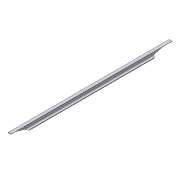
# Autodesk Inventor part: GE-12019-03
Saved by Autodesk Inventor 2012 (Build 160160000, 160)
## iProperties
Created: 2011-06-10
Part Number: GE-12019-03
Document SubType Name: Modeling
Designer: dfoster
Density: 2.71 g/cm^3
Material: Aluminum-6061
Mass: 4063.76 g
Surface Area: 9477.73 cm^2
Volume: 1499.54 cm^3
Description: Channel, Outside
Title: Channel, Outside
Author: dfoster
Autodesk Inventor part; units mm, degrees
ref_plane "YZ Plane" through (0, 0, 0) normal (1, 0, 0) x (0, 1, 0)
ref_plane "XZ Plane" through (0, 0, 0) normal (0, 1, 0) x (-1, 0, 0)
sketch "Sketch1" plane through (0, 0, 0) normal (0, 0, 1) x (1, 0, 0)
  line L0 (0, 0) -> (38.1, 0)
  line L1 (38.1, 76.2) -> (0, 76.2)
  line L2 (0, 76.2) -> (0, 0)
  line L3 (6.5532, 15.2924) -> (6.5532, 60.9076)
  line L4 (12.2838, 67.6723) -> (35.9776, 71.6213)
  line L5 (38.1, 76.2) -> (38.1, 74.1267)
  line L6 (12.2838, 8.5277) -> (35.9776, 4.5787)
  line L7 (38.1, 0) -> (38.1, 2.0733)
  line L8 (24.1307, 69.6468) -> (19.4329, 69.6468)
  arc A0 (38.1, 2.0733) -> (35.9776, 4.5787) centre (35.56, 2.0733) ccw
  arc A1 (35.9776, 71.6213) -> (38.1, 74.1267) centre (35.56, 74.1267) ccw
  arc A2 (6.5532, 15.2924) -> (12.2838, 8.5277) centre (13.4112, 15.2924) ccw
  arc A3 (12.2838, 67.6723) -> (6.5532, 60.9076) centre (13.4112, 60.9076) ccw
  line L9 (0, 91.44) -> (0, -15.24) projected
  line L10 (-7.7119, 0) -> (46.2711, 0) projected
  point P0 (38.1, 71.975)
  dimension "d15" = 76.2
  dimension "d25" = 6.5532
  dimension "d26" = 38.1
  dimension "d28" = 6.5532
  dimension "d29" = 2.54
  dimension "d30" = 6.858
  constraints: 18 end point, 8 point on circle, 8 tangent, 4 centre point, 4 collinear, 2 equal length, 2 equal radius, 2 parallel, 2 point on line, 2 vertical, 1 horizontal, 1 midpoint, 1 perpendicular
  measures "d15" distance between parallel lines of L0 L1
  measures "d25" distance between parallel lines of L2 L3
  measures "d26" distance of L1.start L1.end
  measures "d28" distance between parallel lines of L1 L8
  measures "d29" radius of A0
  measures "d30" radius of A2
extrude "Extrusion1" add sketch "Sketch1" along normal blind 2082.8
sketch "Sketch2" plane through (38.1, 74.1267, 2082.8) normal (1, 0, 0) x (0, 0, -1)
  line L0 (0, 0) -> (959.8939, -1.971)
  line L1 (0, -74.1267) -> (0, -4.2767)
  line L2 (0, -4.2767) -> (241.3, -74.1267)
  line L3 (241.3, -74.1267) -> (0, -74.1267)
  line L4 (2082.8, -74.1267) -> (2082.8, -4.2767)
  line L5 (2082.8, -4.2767) -> (1841.5, -74.1267)
  line L6 (1841.5, -74.1267) -> (2082.8, -74.1267)
  line L7 (2082.8, -74.1267) -> (0, -74.1267) projected
  line L8 (0, -74.1267) -> (0, 2.0733) projected
  line L9 (2082.8, 2.0733) -> (2082.8, -74.1267) projected
  dimension "d19" = 241.3
  dimension "d20" = 69.85
  dimension "d21" = 241.3
  dimension "d31" = 69.85
  constraints: 14 end point, 4 collinear, 2 perpendicular, 1 point on line
  measures "d19" distance from line of L2.end L1
  measures "d20" distance of L4.start L4.end
  measures "d21" distance of L5.end L4.start
  measures "d31" distance of L1.start L1.end
extrude "Extrusion2" cut sketch "Sketch2" against normal blind 304.8
sketch "Sketch3" plane through (6.5532, 60.9076, 2051.9082) normal (1, 0, 0) x (0, 0, -1)
  line L0 (1863.4364, -45.6153) -> (157.58, -45.6153) projected
  circle A0 centre (159.6082, -22.8076) radius 12.7
  line L1 (172.3082, -7.5153) -> (1848.7082, -7.5153)
  line L2 (1848.7082, -7.5153) -> (1848.7082, -42.4403)
  line L3 (1848.7082, -42.4403) -> (172.3082, -42.4403)
  line L4 (172.3082, -42.4403) -> (172.3082, -7.5153)
  line L5 (-30.8918, 8.9424) -> (-30.8918, 15.2924) projected
  line L6 (181.8332, -9.1028) -> (213.5832, -9.1028)
  line L7 (213.5832, -9.1028) -> (213.5832, -40.8528)
  line L8 (213.5832, -40.8528) -> (181.8332, -40.8528)
  line L9 (181.8332, -40.8528) -> (181.8332, -9.1028)
  line L10 (283.4332, -9.1028) -> (315.1832, -9.1028)
  line L11 (315.1832, -9.1028) -> (315.1832, -40.8528)
  line L12 (315.1832, -40.8528) -> (283.4332, -40.8528)
  line L13 (283.4332, -40.8528) -> (283.4332, -9.1028)
  line L14 (385.0332, -9.1028) -> (416.7832, -9.1028)
  line L15 (416.7832, -9.1028) -> (416.7832, -40.8528)
  line L16 (416.7832, -40.8528) -> (385.0332, -40.8528)
  line L17 (385.0332, -40.8528) -> (385.0332, -9.1028)
  line L18 (486.6332, -9.1028) -> (518.3832, -9.1028)
  line L19 (518.3832, -9.1028) -> (518.3832, -40.8528)
  line L20 (518.3832, -40.8528) -> (486.6332, -40.8528)
  line L21 (486.6332, -40.8528) -> (486.6332, -9.1028)
  line L22 (588.2332, -9.1028) -> (619.9832, -9.1028)
  line L23 (619.9832, -9.1028) -> (619.9832, -40.8528)
  line L24 (619.9832, -40.8528) -> (588.2332, -40.8528)
  line L25 (588.2332, -40.8528) -> (588.2332, -9.1028)
  line L26 (689.8332, -9.1028) -> (721.5832, -9.1028)
  line L27 (721.5832, -9.1028) -> (721.5832, -40.8528)
  line L28 (721.5832, -40.8528) -> (689.8332, -40.8528)
  line L29 (689.8332, -40.8528) -> (689.8332, -9.1028)
  line L30 (791.4332, -9.1028) -> (823.1832, -9.1028)
  line L31 (823.1832, -9.1028) -> (823.1832, -40.8528)
  line L32 (823.1832, -40.8528) -> (791.4332, -40.8528)
  line L33 (791.4332, -40.8528) -> (791.4332, -9.1028)
  line L34 (893.0332, -9.1028) -> (924.7832, -9.1028)
  line L35 (924.7832, -9.1028) -> (924.7832, -40.8528)
  line L36 (924.7832, -40.8528) -> (893.0332, -40.8528)
  line L37 (893.0332, -40.8528) -> (893.0332, -9.1028)
  line L38 (994.6332, -9.1028) -> (1026.3832, -9.1028)
  line L39 (1026.3832, -9.1028) -> (1026.3832, -40.8528)
  line L40 (1026.3832, -40.8528) -> (994.6332, -40.8528)
  line L41 (994.6332, -40.8528) -> (994.6332, -9.1028)
  line L42 (1096.2332, -9.1028) -> (1127.9832, -9.1028)
  line L43 (1127.9832, -9.1028) -> (1127.9832, -40.8528)
  line L44 (1127.9832, -40.8528) -> (1096.2332, -40.8528)
  line L45 (1096.2332, -40.8528) -> (1096.2332, -9.1028)
  line L46 (1197.8332, -9.1028) -> (1229.5832, -9.1028)
  line L47 (1229.5832, -9.1028) -> (1229.5832, -40.8528)
  line L48 (1229.5832, -40.8528) -> (1197.8332, -40.8528)
  line L49 (1197.8332, -40.8528) -> (1197.8332, -9.1028)
  line L50 (1299.4332, -9.1028) -> (1331.1832, -9.1028)
  line L51 (1331.1832, -9.1028) -> (1331.1832, -40.8528)
  line L52 (1331.1832, -40.8528) -> (1299.4332, -40.8528)
  line L53 (1299.4332, -40.8528) -> (1299.4332, -9.1028)
  line L54 (1401.0332, -9.1028) -> (1432.7832, -9.1028)
  line L55 (1432.7832, -9.1028) -> (1432.7832, -40.8528)
  line L56 (1432.7832, -40.8528) -> (1401.0332, -40.8528)
  line L57 (1401.0332, -40.8528) -> (1401.0332, -9.1028)
  line L58 (1502.6332, -9.1028) -> (1534.3832, -9.1028)
  line L59 (1534.3832, -9.1028) -> (1534.3832, -40.8528)
  line L60 (1534.3832, -40.8528) -> (1502.6332, -40.8528)
  line L61 (1502.6332, -40.8528) -> (1502.6332, -9.1028)
  line L62 (1604.2332, -9.1028) -> (1635.9832, -9.1028)
  line L63 (1635.9832, -9.1028) -> (1635.9832, -40.8528)
  line L64 (1635.9832, -40.8528) -> (1604.2332, -40.8528)
  line L65 (1604.2332, -40.8528) -> (1604.2332, -9.1028)
  line L66 (1705.8332, -9.1028) -> (1737.5832, -9.1028)
  line L67 (1737.5832, -9.1028) -> (1737.5832, -40.8528)
  line L68 (1737.5832, -40.8528) -> (1705.8332, -40.8528)
  line L69 (1705.8332, -40.8528) -> (1705.8332, -9.1028)
  line L70 (1807.4332, -9.1028) -> (1839.1832, -9.1028)
  line L71 (1839.1832, -9.1028) -> (1839.1832, -40.8528)
  line L72 (1839.1832, -40.8528) -> (1807.4332, -40.8528)
  line L73 (1807.4332, -40.8528) -> (1807.4332, -9.1028)
  line L74 (2051.9082, 15.2924) -> (-30.8918, 15.2924) projected
  line L75 (1010.5082, -7.5153) -> (1010.5082, -42.4403)
  point P0 (2051.9082, -60.9076)
  dimension "d32" = 25.4
  dimension "d33" = 34.925
  dimension "d34" = 3.175
  dimension "d35" = 1676.4
  dimension "d36" = 203.2
  dimension "d37" = 31.75
  dimension "d38" = 1.5875
  dimension "d41" = 101.6
  dimension "d46" = 190.5
  dimension "d47" = 38.1
  dimension "d48" = 9.525
  dimension "d63" = 838.2
  constraints: 146 end point, 4 parallel, 4 perpendicular, 3 horizontal, 2 midpoint, 1 centre point, 128 other
  measures "d32" diameter of A0
  measures "d33" distance between parallel lines of L1 L3
  measures "d34" distance between parallel lines of L0 L3
  measures "d35" distance of L1.start L1.end
  measures "d36" distance between parallel lines of L4 L5
  measures "d37" distance of L6.start L6.end
  measures "d38" distance between parallel lines of L3 L8
  measures "d41" distance of L8.end L13.start
  measures "d46" distance from line of A0.centre L5
  measures "d47" distance from line of A0.centre L74
  measures "d48" distance between parallel lines of L9 L4
  measures "d63" distance between parallel lines of L4 L75
extrude "Extrusion3" cut sketch "Sketch3" against normal blind 25.4 contours A0
hole "Hole1" at (6.5532, 38.1, 1803.4) direction (-1, 0, 0) diameter 3.5719 depth 25.4 tip angle 118
pattern_linear "Rectangular Pattern1" count 2 spacing 711.2 along (0, 0, -1) of "Hole1"
ref_plane "Work Plane1" through (0, 0, 1041.4) normal (0, 0, 1) x (1, 0, 0)
mirror "Mirror1" about plane through (0, 0, 1041.4) normal (0, 0, 1) of "Hole1", "Rectangular Pattern1"
equation "\"d21\" = d19"
equation "\"d31\" = d20"
body "Solid1"
